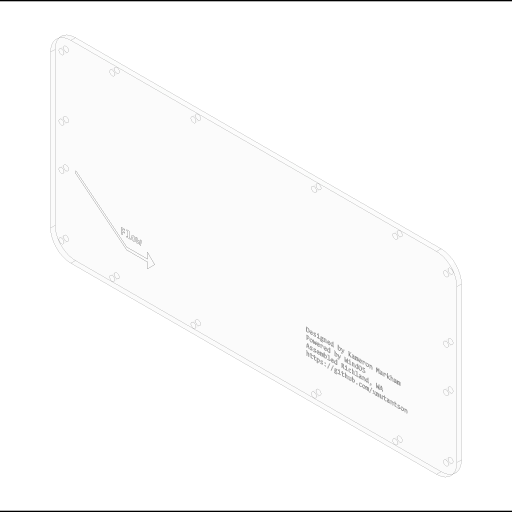
# Autodesk Inventor part: Wind Tunnel Test Section Door Outer
Saved by Autodesk Inventor 2023 (Build 270158000, 158)
## iProperties
Created: 2022-03-08
Part Number: Wind Tunnel Test Section Door Outer
Material: Polycarbonate, Clear
Document SubType Name: Modeling
Designer: kamer
Density: 1.2 g/cm^3
Appearance: Polycarbonate - Clear
Author: kamer
Autodesk Inventor part; units mm, degrees
(part 1 of 3)
ref_plane "YZ Plane" through (0, 0, 0) normal (1, 0, 0) x (0, 1, 0)
ref_plane "XZ Plane" through (0, 0, 0) normal (0, 1, 0) x (-1, 0, 0)
ref_plane "XY Plane" through (0, 0, 0) normal (0, 0, 1) x (1, 0, 0)
sketch "Sketch1" plane through (0, 0, 0) normal (0, 0, 1) x (1, 0, 0)
  line L0 (25.4, 0) -> (482.6, 0)
  line L1 (508, 25.4) -> (508, 215.9)
  line L2 (482.6, 241.3) -> (25.4, 241.3)
  line L3 (0, 215.9) -> (0, 25.4)
  arc A0 (25.4, 241.3) -> (0, 215.9) centre (25.4, 215.9) ccw
  arc A1 (508, 215.9) -> (482.6, 241.3) centre (482.6, 215.9) ccw
  arc A2 (482.6, 0) -> (508, 25.4) centre (482.6, 25.4) ccw
  arc A3 (0, 25.4) -> (25.4, 0) centre (25.4, 25.4) ccw
  point P0 (0, 0)
  point P1 (508, 241.3)
  point P2 (508, 0)
  point P3 (0, 241.3)
  dimension "d0" = 508
  dimension "d1" = 241.3
  dimension "d2" = 25.4
  constraints: 8 end point, 8 point on circle, 8 point on line, 8 tangent, 4 centre point, 3 equal radius, 2 parallel, 1 horizontal, 1 perpendicular
  measures "d0" distance of point (0, 241.3) point (508, 241.3)
  measures "d1" distance of point (508, 241.3) point (508, 0)
  measures "d2" radius of A0
extrude "Extrusion1" add sketch "Sketch1" along normal blind 5.7658
sketch "Sketch2" plane through (0, 0, 5.7658) normal (0, 0, 1) x (1, 0, 0)
  circle A0 centre (13.589, 223.012) radius 3.175
  line L0 (0, 215.9) -> (0, 25.4) projected
  line L1 (482.6, 241.3) -> (25.4, 241.3) projected
  circle A1 centre (13.589, 146.812) radius 3.175
  circle A2 centre (13.589, 94.4626) radius 3.175
  circle A3 centre (13.589, 18.2626) radius 3.175
  circle A4 centre (494.4364, 223.012) radius 3.175
  circle A5 centre (494.4364, 146.812) radius 3.175
  circle A6 centre (494.4364, 94.4626) radius 3.175
  circle A7 centre (494.4364, 18.2626) radius 3.175
  circle A8 centre (77.089, 231.902) radius 3.175
  circle A9 centre (178.689, 231.902) radius 3.175
  circle A10 centre (329.3364, 231.902) radius 3.175
  circle A11 centre (430.9364, 231.902) radius 3.175
  circle A12 centre (77.089, 9.3726) radius 3.175
  circle A13 centre (178.689, 9.3726) radius 3.175
  circle A14 centre (329.3364, 9.3726) radius 3.175
  circle A15 centre (430.9364, 9.3726) radius 3.175
  point P0 (0, 0)
  dimension "d5" = 6.35
  dimension "d6" = 13.589
  dimension "d7" = 18.288
  dimension "d8" = 6.35
  dimension "d9" = 76.2
  dimension "d10" = 13.589
  dimension "d11" = 6.35
  dimension "d12" = 52.3494
  dimension "d13" = 13.589
  dimension "d14" = 6.35
  dimension "d15" = 76.2
  dimension "d16" = 13.589
  dimension "d19" = 480.8474
  dimension "d24" = 6.35
  dimension "d25" = 63.5
  dimension "d26" = 8.89
  dimension "d27" = 6.35
  dimension "d28" = 101.6
  dimension "d29" = 6.35
  dimension "d30" = 150.6474
  dimension "d31" = 6.35
  dimension "d32" = 101.6
  dimension "d33" = 9.398
  dimension "d34" = 9.398
  dimension "d35" = 9.398
  dimension "d38" = 222.5294
  constraints: 16 centre point, 1 horizontal, 1 vertical, 16 other
  measures "d5" diameter of A0
  measures "d6" distance from line of L0 A0.centre
  measures "d7" distance from line of A0.centre L1
  measures "d8" diameter of A1
  measures "d9" distance of A1.centre A0.centre
  measures "d10" distance from line of L0 A1.centre
  measures "d11" diameter of A2
  measures "d12" distance of A2.centre A1.centre
  measures "d13" distance from line of L0 A2.centre
  measures "d14" diameter of A3
  measures "d15" distance of A3.centre A2.centre
  measures "d16" distance from line of L0 A3.centre
  measures "d19" distance of A0.centre A4.centre
  measures "d24" diameter of A8
  measures "d25" horizontal distance of A8.centre A0.centre
  measures "d26" vertical distance of A0.centre A8.centre
  measures "d27" diameter of A9
  measures "d28" distance of A9.centre A8.centre
  measures "d29" diameter of A10
  measures "d30" distance of A10.centre A9.centre
  measures "d31" diameter of A11
  measures "d32" distance of A10.centre A11.centre
  measures "d33" distance from line of L1 A11.centre
  measures "d34" distance from line of L1 A10.centre
  measures "d35" distance from line of L1 A9.centre
  measures "d38" distance of A8.centre A12.centre
extrude "Extrusion2" cut sketch "Sketch2" against normal through all
sketch "Sketch3" plane through (0, 0, 5.7658) normal (0, 0, 1) x (1, 0, 0)
  line L0 (31.75, 101.6) -> (95.25, 50.8) construction
  line L1 (95.25, 50.8) -> (121.1904, 50.8) construction
  line L2 (130.175, 50.8) -> (121.1904, 59.7846)
  line L3 (121.1904, 59.7846) -> (121.1904, 41.8154)
  line L4 (121.1904, 41.8154) -> (130.175, 50.8)
  line L5 (0, 215.9) -> (0, 25.4) projected
  line L6 (25.4, 0) -> (482.6, 0) projected
  line L7 (87.4073, 71.1521) -> (112.3915, 71.1521) construction
  line L8 (112.3915, 71.1521) -> (112.3915, 60.7928) construction
  line L9 (112.3915, 60.7928) -> (87.4073, 60.7928) construction
  line L10 (87.4073, 60.7928) -> (87.4073, 71.1521) construction
  line L11 (319.3804, 78.7378) -> (430.3775, 78.7378) construction
  line L12 (430.3775, 78.7378) -> (430.3775, 29.4798) construction
  line L13 (430.3775, 29.4798) -> (319.3804, 29.4798) construction
  line L14 (319.3804, 29.4798) -> (319.3804, 78.7378) construction
  line L15 (121.1904, 52.3875) -> (95.2986, 52.3875)
  line L16 (95.2986, 52.3875) -> (31.731, 103.2416)
  line L17 (121.1904, 49.2125) -> (95.2014, 49.2125)
  line L18 (95.2014, 49.2125) -> (31.731, 99.9888)
  line L19 (31.731, 99.9888) -> (31.731, 103.2416)
  line L20 (89.9405, 69.3154) -> (89.9405, 67.2124)
  line L21 (89.9405, 67.2124) -> (92.8151, 67.2124)
  line L22 (92.8151, 67.2124) -> (92.8151, 66.0312)
  line L23 (92.8151, 66.0312) -> (89.9405, 66.0312)
  line L24 (89.9405, 66.0312) -> (89.9405, 62.9108)
  line L25 (89.9405, 62.9108) -> (88.4793, 62.9108)
  line L26 (88.4793, 62.9108) -> (88.4793, 70.5308)
  line L27 (88.4793, 70.5308) -> (92.9789, 70.5308)
  line L28 (92.9789, 70.5308) -> (92.9789, 69.3154)
  line L29 (92.9789, 69.3154) -> (89.9405, 69.3154)
  line L30 (96.7002, 70.046) -> (95.0341, 70.046)
  line L31 (95.0341, 70.046) -> (95.0341, 71.1521)
  line L32 (95.0341, 71.1521) -> (98.1613, 71.1521)
  line L33 (98.1613, 71.1521) -> (98.1613, 64.0169)
  line L34 (98.1613, 64.0169) -> (99.8683, 64.0169)
  line L35 (99.8683, 64.0169) -> (99.8683, 62.9108)
  line L36 (99.8683, 62.9108) -> (94.8293, 62.9108)
  line L37 (94.8293, 62.9108) -> (94.8293, 64.0169)
  line L38 (94.8293, 64.0169) -> (96.7002, 64.0169)
  line L39 (96.7002, 64.0169) -> (96.7002, 70.046)
  spline S0 degree 2 poles (106.6895, 65.9151) (106.6895, 65.2186) (106.2934, 64.0579) (105.5492, 63.2317) (104.4636, 62.7742) (103.7671, 62.7742) knots 0 0 0 1 2 3 4 4 4
  spline S1 degree 2 poles (103.7671, 62.7742) (103.1048, 62.7742) (102.0669, 63.1566) (101.3432, 63.9213) (100.9608, 65.0684) (100.9608, 65.8331) knots 0 0 0 1 2 3 4 4 4
  spline S2 degree 2 poles (100.9608, 65.8331) (100.9608, 66.5433) (101.3637, 67.6972) (102.1147, 68.5097) (103.2004, 68.9603) (103.8832, 68.9603) knots 0 0 0 1 2 3 4 4 4
  spline S3 degree 2 poles (103.8832, 68.9603) (104.5455, 68.9603) (105.5902, 68.5712) (106.3071, 67.7996) (106.6895, 66.6662) (106.6895, 65.9151) knots 0 0 0 1 2 3 4 4 4
  spline S4 degree 2 poles (105.2078, 65.8809) (105.2078, 66.8027) (104.5113, 67.7313) (103.8354, 67.7313) knots 0 0 0 1 2 2 2
  spline S5 degree 2 poles (103.8354, 67.7313) (103.4667, 67.7313) (102.9409, 67.4377) (102.5995, 66.9324) (102.4425, 66.2565) (102.4425, 65.8673) knots 0 0 0 1 2 3 4 4 4
  spline S6 degree 2 poles (102.4425, 65.8673) (102.4425, 64.9455) (103.1867, 64.0033) (103.8354, 64.0033) knots 0 0 0 1 2 2 2
  spline S7 degree 2 poles (103.8354, 64.0033) (104.1904, 64.0033) (104.7162, 64.29) (105.0439, 64.7953) (105.2078, 65.4849) (105.2078, 65.8809) knots 0 0 0 1 2 3 4 4 4
  line L40 (112.7868, 62.9108) -> (111.2096, 62.9108)
  line L41 (111.2096, 62.9108) -> (110.5814, 64.7953)
  line L42 (110.5814, 64.7953) -> (110.3902, 65.4508)
  line L43 (110.3902, 65.4508) -> (110.1922, 64.7748)
  line L44 (110.1922, 64.7748) -> (109.5845, 62.9108)
  line L45 (109.5845, 62.9108) -> (108.0004, 62.9108)
  line L46 (108.0004, 62.9108) -> (107.1674, 68.8374)
  line L47 (107.1674, 68.8374) -> (108.5194, 68.8374)
  line L48 (108.5194, 68.8374) -> (108.9427, 65.4781)
  line L49 (108.9427, 65.4781) -> (109.0383, 64.57)
  line L50 (109.0383, 64.57) -> (109.2773, 65.3962)
  line L51 (109.2773, 65.3962) -> (109.8713, 67.1987)
  line L52 (109.8713, 67.1987) -> (110.9569, 67.1987)
  line L53 (110.9569, 67.1987) -> (111.5919, 65.403)
  line L54 (111.5919, 65.403) -> (111.8651, 64.5563)
  line L55 (111.8651, 64.5563) -> (111.9743, 65.4986)
  line L56 (111.9743, 65.4986) -> (112.3362, 68.8374)
  line L57 (112.3362, 68.8374) -> (113.6267, 68.8374)
  line L58 (113.6267, 68.8374) -> (112.7868, 62.9108)
  spline S8 degree 2 poles (323.4726, 75.7927) (323.4726, 75.4285) (323.3588, 74.7594) (323.113, 74.1858) (322.717, 73.717) (322.1389, 73.3801) (321.3787, 73.1981) (320.8916, 73.1981) knots 0 0 0 1 2 3 4 5 6 6 6
  line L59 (320.8916, 73.1981) -> (319.8037, 73.1981)
  line L60 (319.8037, 73.1981) -> (319.8037, 78.2781)
  line L61 (319.8037, 78.2781) -> (321.1147, 78.2781)
  spline S9 degree 2 poles (321.1147, 78.2781) (322.3028, 78.2781) (323.4726, 77.0536) (323.4726, 75.7927) knots 0 0 0 1 2 2 2
  spline S10 degree 2 poles (322.7443, 75.7472) (322.7443, 76.2843) (322.544, 77.0308) (322.1298, 77.4906) (321.5107, 77.6954) (321.0919, 77.6954) knots 0 0 0 1 2 3 4 4 4
  line L62 (321.0919, 77.6954) -> (320.4956, 77.6954)
  line L63 (320.4956, 77.6954) -> (320.4956, 73.7989)
  line L64 (320.4956, 73.7989) -> (321.01, 73.7989)
  spline S11 degree 2 poles (321.01, 73.7989) (322.7443, 73.7989) (322.7443, 75.7472) knots 0 0 0 1 1 1
  spline S12 degree 2 poles (327.6786, 75.3557) (327.6786, 75.2146) (327.6695, 75.0188) (327.665, 74.9324) knots 0 0 0 1 2 2 2
  line L65 (327.665, 74.9324) -> (324.9201, 74.9324)
  spline S13 degree 2 poles (324.9201, 74.9324) (324.9201, 74.336) (325.5893, 73.6942) (326.222, 73.6942) knots 0 0 0 1 2 2 2
  spline S14 degree 2 poles (326.222, 73.6942) (326.3904, 73.6942) (326.7318, 73.7215) (327.055, 73.7671) (327.3463, 73.8262) (327.4692, 73.8626) knots 0 0 0 1 2 3 4 4 4
  line L66 (327.4692, 73.8626) -> (327.4692, 73.3073)
  spline S15 degree 2 poles (327.4692, 73.3073) (327.1916, 73.2299) (326.4951, 73.1298) (326.1219, 73.1298) knots 0 0 0 1 2 2 2
  spline S16 degree 2 poles (326.1219, 73.1298) (325.6211, 73.1298) (324.8974, 73.4029) (324.4376, 73.9173) (324.2146, 74.6683) (324.2146, 75.1417) knots 0 0 0 1 2 3 4 4 4
  spline S17 degree 2 poles (324.2146, 75.1417) (324.2146, 75.556) (324.4513, 76.2888) (324.9065, 76.8442) (325.5665, 77.1719) (325.9853, 77.1719) knots 0 0 0 1 2 3 4 4 4
  spline S18 degree 2 poles (325.9853, 77.1719) (326.395, 77.1719) (327.0277, 76.917) (327.4556, 76.4436) (327.6786, 75.7745) (327.6786, 75.3557) knots 0 0 0 1 2 3 4 4 4
  spline S19 degree 2 poles (326.9731, 75.4513) (326.9867, 75.7107) (326.8593, 76.1432) (326.5998, 76.4573) (326.2129, 76.6302) (325.9534, 76.6302) knots 0 0 0 1 2 3 4 4 4
  spline S20 degree 2 poles (325.9534, 76.6302) (325.7349, 76.6302) (325.3662, 76.4573) (325.1022, 76.1477) (324.9384, 75.7107) (324.9201, 75.4513) knots 0 0 0 1 2 3 4 4 4
  line L67 (324.9201, 75.4513) -> (326.9731, 75.4513)
  spline S21 degree 2 poles (331.8482, 74.2632) (331.8482, 74.0584) (331.7071, 73.7306) (331.4659, 73.4803) (331.1472, 73.3028) (330.7876, 73.1844) (330.4053, 73.1298) (330.2232, 73.1298) knots 0 0 0 1 2 3 4 5 6 6 6
  spline S22 degree 2 poles (330.2232, 73.1298) (329.8272, 73.1298) (329.1626, 73.2026) (328.8439, 73.28) knots 0 0 0 1 2 2 2
  line L68 (328.8439, 73.28) -> (328.8439, 73.9036)
  spline S23 degree 2 poles (328.8439, 73.9036) (329.1853, 73.8035) (329.8636, 73.7033) (330.1959, 73.7033) knots 0 0 0 1 2 2 2
  spline S24 degree 2 poles (330.1959, 73.7033) (330.6829, 73.7033) (331.1472, 73.9673) (331.1472, 74.2086) knots 0 0 0 1 2 2 2
  spline S25 degree 2 poles (331.1472, 74.2086) (331.1472, 74.3133) (331.0744, 74.4817) (330.8787, 74.6319) (330.4735, 74.7958) (330.1185, 74.9005) knots 0 0 0 1 2 3 4 4 4
  spline S26 degree 2 poles (330.1185, 74.9005) (329.8545, 74.9779) (329.4084, 75.1782) (329.0806, 75.4513) (328.894, 75.8154) (328.894, 76.0658) knots 0 0 0 1 2 3 4 4 4
  spline S27 degree 2 poles (328.894, 76.0658) (328.894, 76.2297) (329.0442, 76.6166) (329.4129, 76.9489) (330.032, 77.1719) (330.5009, 77.1719) knots 0 0 0 1 2 3 4 4 4
  spline S28 degree 2 poles (330.5009, 77.1719) (330.7285, 77.1719) (331.2884, 77.1219) (331.5933, 77.0581) knots 0 0 0 1 2 2 2
  line L69 (331.5933, 77.0581) -> (331.5933, 76.4573)
  spline S29 degree 2 poles (331.5933, 76.4573) (331.2747, 76.5347) (330.7011, 76.6075) (330.4918, 76.6075) knots 0 0 0 1 2 2 2
  spline S30 degree 2 poles (330.4918, 76.6075) (330.2414, 76.6075) (329.8954, 76.5301) (329.6815, 76.3935) (329.5859, 76.2115) (329.5859, 76.1068) knots 0 0 0 1 2 3 4 4 4
  spline S31 degree 2 poles (329.5859, 76.1068) (329.5859, 76.0021) (329.6679, 75.8291) (329.8909, 75.6698) (330.2869, 75.5105) (330.6056, 75.4194) knots 0 0 0 1 2 3 4 4 4
  spline S32 degree 2 poles (330.6056, 75.4194) (330.9515, 75.3193) (331.4249, 75.0962) (331.7208, 74.8231) (331.8482, 74.4817) (331.8482, 74.2632) knots 0 0 0 1 2 3 4 4 4
  line L70 (334.4702, 76.5392) -> (333.314, 76.5392)
  line L71 (333.314, 76.5392) -> (333.314, 77.0991)
  line L72 (333.314, 77.0991) -> (335.153, 77.0991)
  line L73 (335.153, 77.0991) -> (335.153, 73.7625)
  line L74 (335.153, 73.7625) -> (336.3137, 73.7625)
  line L75 (336.3137, 73.7625) -> (336.3137, 73.1981)
  line L76 (336.3137, 73.1981) -> (333.1865, 73.1981)
  line L77 (333.1865, 73.1981) -> (333.1865, 73.7625)
  line L78 (333.1865, 73.7625) -> (334.4702, 73.7625)
  line L79 (334.4702, 73.7625) -> (334.4702, 76.5392)
  spline S33 degree 2 poles (334.7069, 78.7378) (334.8207, 78.7378) (335.0119, 78.6559) (335.1575, 78.5102) (335.2395, 78.319) (335.2395, 78.2052) knots 0 0 0 1 2 3 4 4 4
  spline S34 degree 2 poles (335.2395, 78.2052) (335.2395, 78.096) (335.1575, 77.9002) (335.0119, 77.7546) (334.8207, 77.6726) (334.7069, 77.6726) knots 0 0 0 1 2 3 4 4 4
  spline S35 degree 2 poles (334.7069, 77.6726) (334.5931, 77.6726) (334.4019, 77.7546) (334.2562, 77.9002) (334.1743, 78.096) (334.1743, 78.2052) knots 0 0 0 1 2 3 4 4 4
  spline S36 degree 2 poles (334.1743, 78.2052) (334.1743, 78.319) (334.2562, 78.5102) (334.4019, 78.6559) (334.5931, 78.7378) (334.7069, 78.7378) knots 0 0 0 1 2 3 4 4 4
  spline S37 degree 2 poles (340.3286, 76.5483) (340.4378, 76.4117) (340.5562, 76.0521) (340.5562, 75.8428) knots 0 0 0 1 2 2 2
  spline S38 degree 2 poles (340.5562, 75.8428) (340.5562, 75.5378) (340.3331, 75.0371) (339.9325, 74.682) (339.3681, 74.4817) (339.0313, 74.4817) knots 0 0 0 1 2 3 4 4 4
  spline S39 degree 2 poles (339.0313, 74.4817) (338.7854, 74.4817) (338.3576, 74.5864) (338.2347, 74.6638) knots 0 0 0 1 2 2 2
  spline S40 degree 2 poles (338.2347, 74.6638) (338.1573, 74.5545) (338.0571, 74.3634) (338.0571, 74.2405) knots 0 0 0 1 2 2 2
  spline S41 degree 2 poles (338.0571, 74.2405) (338.0571, 74.0948) (338.3394, 73.8991) (338.5761, 73.89) knots 0 0 0 1 2 2 2
  line L80 (338.5761, 73.89) -> (339.6003, 73.8535)
  spline S42 degree 2 poles (339.6003, 73.8535) (339.8916, 73.8444) (340.3877, 73.7124) (340.7382, 73.4621) (340.9385, 73.0979) (340.9385, 72.8567) knots 0 0 0 1 2 3 4 4 4
  spline S43 degree 2 poles (340.9385, 72.8567) (340.9385, 72.5972) (340.7109, 72.1283) (340.2421, 71.7733) (339.5183, 71.5639) (339.0222, 71.5639) knots 0 0 0 1 2 3 4 4 4
  spline S44 degree 2 poles (339.0222, 71.5639) (338.5487, 71.5639) (337.8842, 71.7141) (337.4563, 71.9827) (337.2605, 72.3514) (337.2605, 72.5744) knots 0 0 0 1 2 3 4 4 4
  spline S45 degree 2 poles (337.2605, 72.5744) (337.2605, 72.8612) (337.5246, 73.2891) (337.8022, 73.4848) knots 0 0 0 1 2 2 2
  spline S46 degree 2 poles (337.8022, 73.4848) (337.6975, 73.5303) (337.5519, 73.6715) (337.4563, 73.8399) (337.4108, 74.0265) (337.4108, 74.1176) knots 0 0 0 1 2 3 4 4 4
  spline S47 degree 2 poles (337.4108, 74.1176) (337.4108, 74.3679) (337.6475, 74.7867) (337.8113, 74.9733) knots 0 0 0 1 2 2 2
  spline S48 degree 2 poles (337.8113, 74.9733) (337.7385, 75.0644) (337.6247, 75.2373) (337.5428, 75.4331) (337.5018, 75.6652) (337.5018, 75.8109) knots 0 0 0 1 2 3 4 4 4
  spline S49 degree 2 poles (337.5018, 75.8109) (337.5018, 76.1159) (337.7248, 76.6166) (338.1254, 76.9716) (338.6853, 77.1719) (339.0267, 77.1719) knots 0 0 0 1 2 3 4 4 4
  spline S50 degree 2 poles (339.0267, 77.1719) (339.1724, 77.1719) (339.4364, 77.131) (339.5365, 77.0991) knots 0 0 0 1 2 2 2
  line L81 (339.5365, 77.0991) -> (340.9522, 77.0991)
  line L82 (340.9522, 77.0991) -> (340.9522, 76.5483)
  line L83 (340.9522, 76.5483) -> (340.3286, 76.5483)
  spline S51 degree 2 poles (338.1846, 75.8291) (338.1846, 75.6425) (338.3075, 75.3284) (338.5351, 75.1099) (338.8401, 74.9915) (339.0313, 74.9915) knots 0 0 0 1 2 3 4 4 4
  spline S52 degree 2 poles (339.0313, 74.9915) (339.2315, 74.9915) (339.5456, 75.1281) (339.7596, 75.3602) (339.8734, 75.6652) (339.8734, 75.8291) knots 0 0 0 1 2 3 4 4 4
  spline S53 degree 2 poles (339.8734, 75.8291) (339.8734, 76.0112) (339.7505, 76.3253) (339.5229, 76.5438) (339.2179, 76.6621) (339.0313, 76.6621) knots 0 0 0 1 2 3 4 4 4
  spline S54 degree 2 poles (339.0313, 76.6621) (338.8264, 76.6621) (338.5123, 76.521) (338.2984, 76.2934) (338.1846, 75.9884) (338.1846, 75.8291) knots 0 0 0 1 2 3 4 4 4
  spline S55 degree 2 poles (337.9798, 72.6336) (337.9798, 72.3605) (338.5533, 72.1056) (339.0677, 72.1056) knots 0 0 0 1 2 2 2
  spline S56 degree 2 poles (339.0677, 72.1056) (339.3909, 72.1056) (339.8279, 72.2239) (340.0964, 72.4106) (340.2148, 72.6564) (340.2148, 72.7838) knots 0 0 0 1 2 3 4 4 4
  spline S57 degree 2 poles (340.2148, 72.7838) (340.2148, 73.0205) (339.8279, 73.2481) (339.4273, 73.2663) knots 0 0 0 1 2 2 2
  line L84 (339.4273, 73.2663) -> (338.4076, 73.3028)
  spline S58 degree 2 poles (338.4076, 73.3028) (338.2802, 73.2163) (338.1118, 73.0524) (338.0207, 72.8885) (337.9798, 72.7201) (337.9798, 72.6336) knots 0 0 0 1 2 3 4 4 4
  line L85 (341.899, 77.0991) -> (342.5044, 77.0991)
  line L86 (342.5044, 77.0991) -> (342.5317, 76.4709)
  spline S59 degree 2 poles (342.5317, 76.4709) (342.7001, 76.6712) (343.0188, 76.9398) (343.3283, 77.1036) (343.647, 77.1719) (343.8199, 77.1719) knots 0 0 0 1 2 3 4 4 4
  spline S60 degree 2 poles (343.8199, 77.1719) (344.4208, 77.1719) (345.0399, 76.4618) (345.0399, 75.7472) knots 0 0 0 1 2 2 2
  line L87 (345.0399, 75.7472) -> (345.0399, 73.1981)
  line L88 (345.0399, 73.1981) -> (344.3616, 73.1981)
  line L89 (344.3616, 73.1981) -> (344.3616, 75.6925)
  spline S61 degree 2 poles (344.3616, 75.6925) (344.3616, 76.1477) (344.0202, 76.5893) (343.6834, 76.5893) knots 0 0 0 1 2 2 2
  spline S62 degree 2 poles (343.6834, 76.5893) (343.5559, 76.5893) (343.3192, 76.5164) (343.0643, 76.3344) (342.7639, 76.0203) (342.5772, 75.7881) knots 0 0 0 1 2 3 4 4 4
  line L90 (342.5772, 75.7881) -> (342.5772, 73.1981)
  line L91 (342.5772, 73.1981) -> (341.899, 73.1981)
  line L92 (341.899, 73.1981) -> (341.899, 77.0991)
  spline S63 degree 2 poles (349.5736, 75.3557) (349.5736, 75.2146) (349.5645, 75.0188) (349.56, 74.9324) knots 0 0 0 1 2 2 2
  line L93 (349.56, 74.9324) -> (346.8151, 74.9324)
  spline S64 degree 2 poles (346.8151, 74.9324) (346.8151, 74.336) (347.4843, 73.6942) (348.117, 73.6942) knots 0 0 0 1 2 2 2
  spline S65 degree 2 poles (348.117, 73.6942) (348.2854, 73.6942) (348.6268, 73.7215) (348.95, 73.7671) (349.2413, 73.8262) (349.3642, 73.8626) knots 0 0 0 1 2 3 4 4 4
  line L94 (349.3642, 73.8626) -> (349.3642, 73.3073)
  spline S66 degree 2 poles (349.3642, 73.3073) (349.0866, 73.2299) (348.3901, 73.1298) (348.0168, 73.1298) knots 0 0 0 1 2 2 2
  spline S67 degree 2 poles (348.0168, 73.1298) (347.5161, 73.1298) (346.7924, 73.4029) (346.3326, 73.9173) (346.1096, 74.6683) (346.1096, 75.1417) knots 0 0 0 1 2 3 4 4 4
  spline S68 degree 2 poles (346.1096, 75.1417) (346.1096, 75.556) (346.3463, 76.2888) (346.8015, 76.8442) (347.4615, 77.1719) (347.8803, 77.1719) knots 0 0 0 1 2 3 4 4 4
  spline S69 degree 2 poles (347.8803, 77.1719) (348.29, 77.1719) (348.9227, 76.917) (349.3506, 76.4436) (349.5736, 75.7745) (349.5736, 75.3557) knots 0 0 0 1 2 3 4 4 4
  spline S70 degree 2 poles (348.8681, 75.4513) (348.8817, 75.7107) (348.7543, 76.1432) (348.4948, 76.4573) (348.1079, 76.6302) (347.8484, 76.6302) knots 0 0 0 1 2 3 4 4 4
  spline S71 degree 2 poles (347.8484, 76.6302) (347.6299, 76.6302) (347.2612, 76.4573) (346.9972, 76.1477) (346.8333, 75.7107) (346.8151, 75.4513) knots 0 0 0 1 2 3 4 4 4
  line L95 (346.8151, 75.4513) -> (348.8681, 75.4513)
  spline S72 degree 2 poles (350.4567, 75.0689) (350.4567, 75.5651) (350.7298, 76.3389) (351.2305, 76.8715) (351.9315, 77.1492) (352.364, 77.1492) knots 0 0 0 1 2 3 4 4 4
  spline S73 degree 2 poles (352.364, 77.1492) (352.5506, 77.1492) (352.9148, 77.1036) (353.0877, 77.0536) knots 0 0 0 1 2 2 2
  line L96 (353.0877, 77.0536) -> (353.0877, 78.6923)
  line L97 (353.0877, 78.6923) -> (353.766, 78.6923)
  line L98 (353.766, 78.6923) -> (353.766, 73.1981)
  line L99 (353.766, 73.1981) -> (353.1606, 73.1981)
  line L100 (353.1606, 73.1981) -> (353.1378, 73.94)
  spline S74 degree 2 poles (353.1378, 73.94) (352.8556, 73.5258) (352.1956, 73.1298) (351.8086, 73.1298) knots 0 0 0 1 2 2 2
  spline S75 degree 2 poles (351.8086, 73.1298) (351.4763, 73.1298) (350.9665, 73.4074) (350.6297, 73.9173) (350.4567, 74.6319) (350.4567, 75.0689) knots 0 0 0 1 2 3 4 4 4
  spline S76 degree 2 poles (351.1486, 75.1099) (351.1486, 74.4043) (351.5628, 73.7079) (351.9452, 73.7079) knots 0 0 0 1 2 2 2
  spline S77 degree 2 poles (351.9452, 73.7079) (352.2001, 73.7079) (352.7737, 74.1676) (353.0877, 74.6183) knots 0 0 0 1 2 2 2
  line L101 (353.0877, 74.6183) -> (353.0877, 76.43)
  spline S78 degree 2 poles (353.0877, 76.43) (352.9193, 76.5073) (352.5187, 76.5893) (352.3185, 76.5893) knots 0 0 0 1 2 2 2
  spline S79 degree 2 poles (352.3185, 76.5893) (351.7677, 76.5893) (351.1486, 75.8746) (351.1486, 75.1099) knots 0 0 0 1 2 2 2
  spline S80 degree 2 poles (362.7516, 75.2191) (362.7516, 74.7366) (362.483, 73.9673) (361.9914, 73.4348) (361.2813, 73.1525) (360.8398, 73.1525) knots 0 0 0 1 2 3 4 4 4
  spline S81 degree 2 poles (360.8398, 73.1525) (360.4938, 73.1525) (359.77, 73.2845) (359.415, 73.4302) knots 0 0 0 1 2 2 2
  line L102 (359.415, 73.4302) -> (359.415, 78.6923)
  line L103 (359.415, 78.6923) -> (360.0932, 78.6923)
  line L104 (360.0932, 78.6923) -> (360.0932, 77.181)
  line L105 (360.0932, 77.181) -> (360.0614, 76.4573)
  spline S82 degree 2 poles (360.0614, 76.4573) (360.3527, 76.8487) (361.0173, 77.1719) (361.3996, 77.1719) knots 0 0 0 1 2 2 2
  spline S83 degree 2 poles (361.3996, 77.1719) (361.7319, 77.1719) (362.2372, 76.8943) (362.5786, 76.3844) (362.7516, 75.6652) (362.7516, 75.2191) knots 0 0 0 1 2 3 4 4 4
  spline S84 degree 2 poles (362.0597, 75.1873) (362.0597, 75.4968) (361.9686, 76.0066) (361.7775, 76.3753) (361.4725, 76.5802) (361.2631, 76.5802) knots 0 0 0 1 2 3 4 4 4
  spline S85 degree 2 poles (361.2631, 76.5802) (361.1356, 76.5802) (360.8716, 76.4982) (360.5848, 76.3071) (360.2708, 75.993) (360.0932, 75.7608) knots 0 0 0 1 2 3 4 4 4
  line L106 (360.0932, 75.7608) -> (360.0932, 73.8672)
  spline S86 degree 2 poles (360.0932, 73.8672) (360.2935, 73.7898) (360.7032, 73.6988) (360.8898, 73.6988) knots 0 0 0 1 2 2 2
  spline S87 degree 2 poles (360.8898, 73.6988) (361.122, 73.6988) (361.5453, 73.8444) (361.8685, 74.1904) (362.0597, 74.7639) (362.0597, 75.1873) knots 0 0 0 1 2 3 4 4 4
  line L107 (367.2671, 77.0991) -> (365.938, 73.6123)
  spline S88 degree 2 poles (365.938, 73.6123) (365.7286, 73.0797) (365.2916, 72.3104) (364.7681, 71.8143) (364.149, 71.5821) (363.7621, 71.5821) knots 0 0 0 1 2 3 4 4 4
  spline S89 degree 2 poles (363.7621, 71.5821) (363.662, 71.5821) (363.4981, 71.5912) (363.4025, 71.6003) knots 0 0 0 1 2 2 2
  line L108 (363.4025, 71.6003) -> (363.4025, 72.2148)
  spline S90 degree 2 poles (363.4025, 72.2148) (363.4844, 72.2012) (363.6893, 72.183) (363.8031, 72.183) knots 0 0 0 1 2 2 2
  spline S91 degree 2 poles (363.8031, 72.183) (363.9897, 72.183) (364.3129, 72.2922) (364.5997, 72.5335) (364.8637, 72.9249) (364.9866, 73.1981) knots 0 0 0 1 2 3 4 4 4
  line L109 (364.9866, 73.1981) -> (363.4298, 77.0991)
  line L110 (363.4298, 77.0991) -> (364.1991, 77.0991)
  line L111 (364.1991, 77.0991) -> (365.1869, 74.5181)
  line L112 (365.1869, 74.5181) -> (365.3872, 73.9127)
  line L113 (365.3872, 73.9127) -> (365.6102, 74.5363)
  line L114 (365.6102, 74.5363) -> (366.5206, 77.0991)
  line L115 (366.5206, 77.0991) -> (367.2671, 77.0991)
  line L116 (375.9978, 73.1981) -> (375.1284, 73.1981)
  line L117 (375.1284, 73.1981) -> (373.2257, 75.688)
  line L118 (373.2257, 75.688) -> (373.2257, 73.1981)
  line L119 (373.2257, 73.1981) -> (372.5338, 73.1981)
  line L120 (372.5338, 73.1981) -> (372.5338, 78.2781)
  line L121 (372.5338, 78.2781) -> (373.2257, 78.2781)
  line L122 (373.2257, 78.2781) -> (373.2257, 75.9156)
  line L123 (373.2257, 75.9156) -> (375.0874, 78.2781)
  line L124 (375.0874, 78.2781) -> (375.9068, 78.2781)
  line L125 (375.9068, 78.2781) -> (373.9039, 75.8655)
  line L126 (373.9039, 75.8655) -> (375.9978, 73.1981)
  line L127 (379.4391, 73.1981) -> (379.4255, 73.7215)
  spline S92 degree 2 poles (379.4255, 73.7215) (379.1068, 73.4074) (378.4468, 73.1298) (378.0872, 73.1298) knots 0 0 0 1 2 2 2
  spline S93 degree 2 poles (378.0872, 73.1298) (377.7503, 73.1298) (377.2769, 73.3028) (376.9719, 73.5986) (376.8263, 74.0038) (376.8263, 74.2405) knots 0 0 0 1 2 3 4 4 4
  spline S94 degree 2 poles (376.8263, 74.2405) (376.8263, 74.8277) (377.7003, 75.4922) (378.556, 75.4922) knots 0 0 0 1 2 2 2
  line L128 (378.556, 75.4922) -> (379.3663, 75.4922)
  line L129 (379.3663, 75.4922) -> (379.3663, 75.8336)
  spline S95 degree 2 poles (379.3663, 75.8336) (379.3663, 76.1796) (378.9247, 76.5984) (378.4695, 76.5984) knots 0 0 0 1 2 2 2
  spline S96 degree 2 poles (378.4695, 76.5984) (378.1372, 76.5984) (377.4954, 76.4527) (377.154, 76.3162) knots 0 0 0 1 2 2 2
  line L130 (377.154, 76.3162) -> (377.154, 76.9261)
  spline S97 degree 2 poles (377.154, 76.9261) (377.2815, 76.9716) (377.5956, 77.0627) (377.9461, 77.131) (378.3284, 77.1719) (378.5196, 77.1719) knots 0 0 0 1 2 3 4 4 4
  spline S98 degree 2 poles (378.5196, 77.1719) (378.8747, 77.1719) (379.4437, 77.0172) (379.8351, 76.6985) (380.0445, 76.216) (380.0445, 75.8883) knots 0 0 0 1 2 3 4 4 4
  line L131 (380.0445, 75.8883) -> (380.0445, 73.1981)
  line L132 (380.0445, 73.1981) -> (379.4391, 73.1981)
  line L133 (379.3663, 74.9733) -> (378.506, 74.9733)
  spline S99 degree 2 poles (378.506, 74.9733) (378.251, 74.9733) (377.8869, 74.8732) (377.6547, 74.6865) (377.5409, 74.4271) (377.5409, 74.2632) knots 0 0 0 1 2 3 4 4 4
  spline S100 degree 2 poles (377.5409, 74.2632) (377.5409, 74.1494) (377.6092, 73.9446) (377.7685, 73.7853) (378.0143, 73.6942) (378.1964, 73.6942) knots 0 0 0 1 2 3 4 4 4
  spline S101 degree 2 poles (378.1964, 73.6942) (378.4286, 73.6942) (379.0294, 73.9764) (379.3663, 74.2814) knots 0 0 0 1 2 2 2
  line L134 (379.3663, 74.2814) -> (379.3663, 74.9733)
  line L135 (384.0958, 73.1981) -> (384.0958, 76.0021)
  spline S102 degree 2 poles (384.0958, 76.0021) (384.0958, 76.1841) (384.0685, 76.4163) (384.0138, 76.5529) (383.9319, 76.6075) (383.8682, 76.6075) knots 0 0 0 1 2 3 4 4 4
  spline S103 degree 2 poles (383.8682, 76.6075) (383.7953, 76.6075) (383.6724, 76.5164) (383.5313, 76.3025) (383.3629, 75.9565) (383.2446, 75.7062) knots 0 0 0 1 2 3 4 4 4
  line L136 (383.2446, 75.7062) -> (383.2446, 73.1981)
  line L137 (383.2446, 73.1981) -> (382.5663, 73.1981)
  line L138 (382.5663, 73.1981) -> (382.5663, 75.9292)
  spline S104 degree 2 poles (382.5663, 75.9292) (382.5663, 76.1432) (382.539, 76.4072) (382.4844, 76.5529) (382.3979, 76.6075) (382.3342, 76.6075) knots 0 0 0 1 2 3 4 4 4
  spline S105 degree 2 poles (382.3342, 76.6075) (382.2704, 76.6075) (382.1521, 76.5301) (382.011, 76.3298) (381.8334, 75.9793) (381.7151, 75.7062) knots 0 0 0 1 2 3 4 4 4
  line L139 (381.7151, 75.7062) -> (381.7151, 73.1981)
  line L140 (381.7151, 73.1981) -> (381.0368, 73.1981)
  line L141 (381.0368, 73.1981) -> (381.0368, 77.0991)
  line L142 (381.0368, 77.0991) -> (381.6013, 77.0991)
  line L143 (381.6013, 77.0991) -> (381.6332, 76.3571)
  spline S106 degree 2 poles (381.6332, 76.3571) (381.7379, 76.5802) (381.929, 76.8897) (382.1293, 77.0809) (382.3615, 77.1719) (382.498, 77.1719) knots 0 0 0 1 2 3 4 4 4
  spline S107 degree 2 poles (382.498, 77.1719) (382.8167, 77.1719) (383.1444, 76.7577) (383.1444, 76.3253) knots 0 0 0 1 2 2 2
  spline S108 degree 2 poles (383.1444, 76.3253) (383.2355, 76.5301) (383.4175, 76.8442) (383.6224, 77.0581) (383.8727, 77.1719) (384.0366, 77.1719) knots 0 0 0 1 2 3 4 4 4
  spline S109 degree 2 poles (384.0366, 77.1719) (384.774, 77.1719) (384.774, 76.0385) knots 0 0 0 1 1 1
  line L144 (384.774, 76.0385) -> (384.774, 73.1981)
  line L145 (384.774, 73.1981) -> (384.0958, 73.1981)
  spline S110 degree 2 poles (388.9846, 75.3557) (388.9846, 75.2146) (388.9755, 75.0188) (388.9709, 74.9324) knots 0 0 0 1 2 2 2
  line L146 (388.9709, 74.9324) -> (386.2261, 74.9324)
  spline S111 degree 2 poles (386.2261, 74.9324) (386.2261, 74.336) (386.8952, 73.6942) (387.528, 73.6942) knots 0 0 0 1 2 2 2
  spline S112 degree 2 poles (387.528, 73.6942) (387.6964, 73.6942) (388.0378, 73.7215) (388.361, 73.7671) (388.6523, 73.8262) (388.7752, 73.8626) knots 0 0 0 1 2 3 4 4 4
  line L147 (388.7752, 73.8626) -> (388.7752, 73.3073)
  spline S113 degree 2 poles (388.7752, 73.3073) (388.4975, 73.2299) (387.8011, 73.1298) (387.4278, 73.1298) knots 0 0 0 1 2 2 2
  spline S114 degree 2 poles (387.4278, 73.1298) (386.9271, 73.1298) (386.2033, 73.4029) (385.7436, 73.9173) (385.5205, 74.6683) (385.5205, 75.1417) knots 0 0 0 1 2 3 4 4 4
  spline S115 degree 2 poles (385.5205, 75.1417) (385.5205, 75.556) (385.7572, 76.2888) (386.2124, 76.8442) (386.8725, 77.1719) (387.2913, 77.1719) knots 0 0 0 1 2 3 4 4 4
  spline S116 degree 2 poles (387.2913, 77.1719) (387.7009, 77.1719) (388.3337, 76.917) (388.7615, 76.4436) (388.9846, 75.7745) (388.9846, 75.3557) knots 0 0 0 1 2 3 4 4 4
  spline S117 degree 2 poles (388.279, 75.4513) (388.2927, 75.7107) (388.1652, 76.1432) (387.9058, 76.4573) (387.5189, 76.6302) (387.2594, 76.6302) knots 0 0 0 1 2 3 4 4 4
  spline S118 degree 2 poles (387.2594, 76.6302) (387.0409, 76.6302) (386.6722, 76.4573) (386.4082, 76.1477) (386.2443, 75.7107) (386.2261, 75.4513) knots 0 0 0 1 2 3 4 4 4
  line L148 (386.2261, 75.4513) -> (388.279, 75.4513)
  line L149 (390.2273, 77.0991) -> (390.8463, 77.0991)
  line L150 (390.8463, 77.0991) -> (390.8646, 76.3799)
  spline S119 degree 2 poles (390.8646, 76.3799) (391.2105, 76.7987) (391.8796, 77.1719) (392.2256, 77.1719) knots 0 0 0 1 2 2 2
  spline S120 degree 2 poles (392.2256, 77.1719) (392.831, 77.1719) (393.4546, 76.3844) (393.4319, 75.6106) knots 0 0 0 1 2 2 2
  line L151 (393.4319, 75.6106) -> (392.7491, 75.6106)
  spline S121 degree 2 poles (392.7491, 75.6106) (392.7627, 76.125) (392.4395, 76.5893) (392.1255, 76.5893) knots 0 0 0 1 2 2 2
  spline S122 degree 2 poles (392.1255, 76.5893) (391.9889, 76.5893) (391.7158, 76.4937) (391.4244, 76.2752) (391.0967, 75.9429) (390.9101, 75.7016) knots 0 0 0 1 2 3 4 4 4
  line L152 (390.9101, 75.7016) -> (390.9101, 73.1981)
  line L153 (390.9101, 73.1981) -> (390.2273, 73.1981)
  line L154 (390.2273, 73.1981) -> (390.2273, 77.0991)
  spline S123 degree 2 poles (397.8427, 75.1827) (397.8427, 74.7275) (397.5878, 73.9673) (397.1053, 73.4302) (396.4134, 73.1298) (395.9719, 73.1298) knots 0 0 0 1 2 3 4 4 4
  spline S124 degree 2 poles (395.9719, 73.1298) (395.5531, 73.1298) (394.8885, 73.3892) (394.4287, 73.8945) (394.1829, 74.641) (394.1829, 75.1281) knots 0 0 0 1 2 3 4 4 4
  spline S125 degree 2 poles (394.1829, 75.1281) (394.1829, 75.5833) (394.4379, 76.3344) (394.9204, 76.8715) (395.6123, 77.1719) (396.0538, 77.1719) knots 0 0 0 1 2 3 4 4 4
  spline S126 degree 2 poles (396.0538, 77.1719) (396.4726, 77.1719) (397.1372, 76.9125) (397.5969, 76.4117) (397.8427, 75.6652) (397.8427, 75.1827) knots 0 0 0 1 2 3 4 4 4
  spline S127 degree 2 poles (397.1508, 75.1509) (397.1508, 75.515) (396.9915, 76.0521) (396.6956, 76.4163) (396.2723, 76.5984) (396.0128, 76.5984) knots 0 0 0 1 2 3 4 4 4
  spline S128 degree 2 poles (396.0128, 76.5984) (395.7079, 76.5984) (395.28, 76.3617) (395.0023, 75.9657) (394.8748, 75.4422) (394.8748, 75.1509) knots 0 0 0 1 2 3 4 4 4
  spline S129 degree 2 poles (394.8748, 75.1509) (394.8748, 74.7912) (395.0342, 74.2496) (395.33, 73.8854) (395.7488, 73.7033) (396.0128, 73.7033) knots 0 0 0 1 2 3 4 4 4
  spline S130 degree 2 poles (396.0128, 73.7033) (396.3178, 73.7033) (396.7457, 73.94) (397.0234, 74.336) (397.1508, 74.8595) (397.1508, 75.1509) knots 0 0 0 1 2 3 4 4 4
  line L155 (398.826, 77.0991) -> (399.4314, 77.0991)
  line L156 (399.4314, 77.0991) -> (399.4587, 76.4709)
  spline S131 degree 2 poles (399.4587, 76.4709) (399.6271, 76.6712) (399.9457, 76.9398) (400.2553, 77.1036) (400.5739, 77.1719) (400.7469, 77.1719) knots 0 0 0 1 2 3 4 4 4
  spline S132 degree 2 poles (400.7469, 77.1719) (401.3477, 77.1719) (401.9668, 76.4618) (401.9668, 75.7472) knots 0 0 0 1 2 2 2
  line L157 (401.9668, 75.7472) -> (401.9668, 73.1981)
  line L158 (401.9668, 73.1981) -> (401.2886, 73.1981)
  line L159 (401.2886, 73.1981) -> (401.2886, 75.6925)
  spline S133 degree 2 poles (401.2886, 75.6925) (401.2886, 76.1477) (400.9472, 76.5893) (400.6103, 76.5893) knots 0 0 0 1 2 2 2
  spline S134 degree 2 poles (400.6103, 76.5893) (400.4829, 76.5893) (400.2462, 76.5164) (399.9913, 76.3344) (399.6908, 76.0203) (399.5042, 75.7881) knots 0 0 0 1 2 3 4 4 4
  line L160 (399.5042, 75.7881) -> (399.5042, 73.1981)
  line L161 (399.5042, 73.1981) -> (398.826, 73.1981)
  line L162 (398.826, 73.1981) -> (398.826, 77.0991)
  line L163 (411.1481, 73.1981) -> (410.4699, 73.1981)
  line L164 (410.4699, 73.1981) -> (410.3698, 76.3708)
  line L165 (410.3698, 76.3708) -> (410.3288, 77.5816)
  line L166 (410.3288, 77.5816) -> (410.0921, 76.876)
  line L167 (410.0921, 76.876) -> (409.341, 74.855)
  line L168 (409.341, 74.855) -> (408.8631, 74.855)
  line L169 (408.8631, 74.855) -> (408.1484, 76.7987)
  line L170 (408.1484, 76.7987) -> (407.9162, 77.5816)
  line L171 (407.9162, 77.5816) -> (407.898, 76.3162)
  line L172 (407.898, 76.3162) -> (407.807, 73.1981)
  line L173 (407.807, 73.1981) -> (407.1561, 73.1981)
  line L174 (407.1561, 73.1981) -> (407.4064, 78.2781)
  line L175 (407.4064, 78.2781) -> (408.2258, 78.2781)
  line L176 (408.2258, 78.2781) -> (408.9086, 76.3662)
  line L177 (408.9086, 76.3662) -> (409.1271, 75.7198)
  line L178 (409.1271, 75.7198) -> (409.341, 76.3662)
  line L179 (409.341, 76.3662) -> (410.0602, 78.2781)
  line L180 (410.0602, 78.2781) -> (410.9023, 78.2781)
  line L181 (410.9023, 78.2781) -> (411.1481, 73.1981)
  line L182 (414.4711, 73.1981) -> (414.4574, 73.7215)
  spline S135 degree 2 poles (414.4574, 73.7215) (414.1388, 73.4074) (413.4787, 73.1298) (413.1191, 73.1298) knots 0 0 0 1 2 2 2
  spline S136 degree 2 poles (413.1191, 73.1298) (412.7823, 73.1298) (412.3089, 73.3028) (412.0039, 73.5986) (411.8582, 74.0038) (411.8582, 74.2405) knots 0 0 0 1 2 3 4 4 4
  spline S137 degree 2 poles (411.8582, 74.2405) (411.8582, 74.8277) (412.7322, 75.4922) (413.588, 75.4922) knots 0 0 0 1 2 2 2
  line L183 (413.588, 75.4922) -> (414.3982, 75.4922)
  line L184 (414.3982, 75.4922) -> (414.3982, 75.8336)
  spline S138 degree 2 poles (414.3982, 75.8336) (414.3982, 76.1796) (413.9567, 76.5984) (413.5015, 76.5984) knots 0 0 0 1 2 2 2
  spline S139 degree 2 poles (413.5015, 76.5984) (413.1692, 76.5984) (412.5274, 76.4527) (412.186, 76.3162) knots 0 0 0 1 2 2 2
  line L185 (412.186, 76.3162) -> (412.186, 76.9261)
  spline S140 degree 2 poles (412.186, 76.9261) (412.3134, 76.9716) (412.6275, 77.0627) (412.978, 77.131) (413.3604, 77.1719) (413.5516, 77.1719) knots 0 0 0 1 2 3 4 4 4
  spline S141 degree 2 poles (413.5516, 77.1719) (413.9066, 77.1719) (414.4756, 77.0172) (414.8671, 76.6985) (415.0765, 76.216) (415.0765, 75.8883) knots 0 0 0 1 2 3 4 4 4
  line L186 (415.0765, 75.8883) -> (415.0765, 73.1981)
  line L187 (415.0765, 73.1981) -> (414.4711, 73.1981)
  line L188 (414.3982, 74.9733) -> (413.5379, 74.9733)
  spline S142 degree 2 poles (413.5379, 74.9733) (413.283, 74.9733) (412.9189, 74.8732) (412.6867, 74.6865) (412.5729, 74.4271) (412.5729, 74.2632) knots 0 0 0 1 2 3 4 4 4
  spline S143 degree 2 poles (412.5729, 74.2632) (412.5729, 74.1494) (412.6412, 73.9446) (412.8005, 73.7853) (413.0463, 73.6942) (413.2284, 73.6942) knots 0 0 0 1 2 3 4 4 4
  spline S144 degree 2 poles (413.2284, 73.6942) (413.4605, 73.6942) (414.0614, 73.9764) (414.3982, 74.2814) knots 0 0 0 1 2 2 2
  line L189 (414.3982, 74.2814) -> (414.3982, 74.9733)
  line L190 (416.5013, 77.0991) -> (417.1203, 77.0991)
  line L191 (417.1203, 77.0991) -> (417.1385, 76.3799)
  spline S145 degree 2 poles (417.1385, 76.3799) (417.4845, 76.7987) (418.1536, 77.1719) (418.4996, 77.1719) knots 0 0 0 1 2 2 2
  spline S146 degree 2 poles (418.4996, 77.1719) (419.105, 77.1719) (419.7286, 76.3844) (419.7058, 75.6106) knots 0 0 0 1 2 2 2
  line L192 (419.7058, 75.6106) -> (419.0231, 75.6106)
  spline S147 degree 2 poles (419.0231, 75.6106) (419.0367, 76.125) (418.7135, 76.5893) (418.3994, 76.5893) knots 0 0 0 1 2 2 2
  spline S148 degree 2 poles (418.3994, 76.5893) (418.2629, 76.5893) (417.9898, 76.4937) (417.6984, 76.2752) (417.3707, 75.9429) (417.1841, 75.7016) knots 0 0 0 1 2 3 4 4 4
  line L193 (417.1841, 75.7016) -> (417.1841, 73.1981)
  line L194 (417.1841, 73.1981) -> (416.5013, 73.1981)
  line L195 (416.5013, 73.1981) -> (416.5013, 77.0991)
  line L196 (424.226, 73.1981) -> (423.2974, 73.1981)
  line L197 (423.2974, 73.1981) -> (421.4811, 75.292)
  line L198 (421.4811, 75.292) -> (421.4811, 73.1981)
  line L199 (421.4811, 73.1981) -> (420.8029, 73.1981)
  line L200 (420.8029, 73.1981) -> (420.8029, 78.6923)
  line L201 (420.8029, 78.6923) -> (421.4811, 78.6923)
  line L202 (421.4811, 78.6923) -> (421.4811, 75.3193)
  line L203 (421.4811, 75.3193) -> (423.2336, 77.0991)
  line L204 (423.2336, 77.0991) -> (424.1258, 77.0991)
  line L205 (424.1258, 77.0991) -> (422.2959, 75.3011)
  line L206 (422.2959, 75.3011) -> (424.226, 73.1981)
  line L207 (428.2408, 73.1981) -> (427.5625, 73.1981)
  line L208 (427.5625, 73.1981) -> (427.5625, 75.6925)
  spline S149 degree 2 poles (427.5625, 75.6925) (427.5625, 76.1432) (427.2257, 76.5893) (426.9116, 76.5893) knots 0 0 0 1 2 2 2
  spline S150 degree 2 poles (426.9116, 76.5893) (426.7751, 76.5893) (426.5384, 76.5164) (426.2789, 76.3344) (425.9785, 76.0203) (425.7782, 75.7881) knots 0 0 0 1 2 3 4 4 4
  line L209 (425.7782, 75.7881) -> (425.7782, 73.1981)
  line L210 (425.7782, 73.1981) -> (425.0999, 73.1981)
  line L211 (425.0999, 73.1981) -> (425.0999, 78.6923)
  line L212 (425.0999, 78.6923) -> (425.7782, 78.6923)
  line L213 (425.7782, 78.6923) -> (425.7782, 77.1036)
  line L214 (425.7782, 77.1036) -> (425.7554, 76.4891)
  spline S151 degree 2 poles (425.7554, 76.4891) (425.9147, 76.6803) (426.2197, 76.9398) (426.5293, 77.1036) (426.8479, 77.1719) (427.0209, 77.1719) knots 0 0 0 1 2 3 4 4 4
  spline S152 degree 2 poles (427.0209, 77.1719) (427.6035, 77.1719) (428.2408, 76.4618) (428.2408, 75.7472) knots 0 0 0 1 2 2 2
  line L215 (428.2408, 75.7472) -> (428.2408, 73.1981)
  line L216 (431.9871, 73.1981) -> (431.9734, 73.7215)
  spline S153 degree 2 poles (431.9734, 73.7215) (431.6548, 73.4074) (430.9947, 73.1298) (430.6351, 73.1298) knots 0 0 0 1 2 2 2
  spline S154 degree 2 poles (430.6351, 73.1298) (430.2983, 73.1298) (429.8249, 73.3028) (429.5199, 73.5986) (429.3742, 74.0038) (429.3742, 74.2405) knots 0 0 0 1 2 3 4 4 4
  spline S155 degree 2 poles (429.3742, 74.2405) (429.3742, 74.8277) (430.2482, 75.4922) (431.104, 75.4922) knots 0 0 0 1 2 2 2
  line L217 (431.104, 75.4922) -> (431.9142, 75.4922)
  line L218 (431.9142, 75.4922) -> (431.9142, 75.8336)
  spline S156 degree 2 poles (431.9142, 75.8336) (431.9142, 76.1796) (431.4727, 76.5984) (431.0175, 76.5984) knots 0 0 0 1 2 2 2
  spline S157 degree 2 poles (431.0175, 76.5984) (430.6852, 76.5984) (430.0434, 76.4527) (429.702, 76.3162) knots 0 0 0 1 2 2 2
  line L219 (429.702, 76.3162) -> (429.702, 76.9261)
  spline S158 degree 2 poles (429.702, 76.9261) (429.8294, 76.9716) (430.1435, 77.0627) (430.494, 77.131) (430.8764, 77.1719) (431.0676, 77.1719) knots 0 0 0 1 2 3 4 4 4
  spline S159 degree 2 poles (431.0676, 77.1719) (431.4226, 77.1719) (431.9916, 77.0172) (432.3831, 76.6985) (432.5925, 76.216) (432.5925, 75.8883) knots 0 0 0 1 2 3 4 4 4
  line L220 (432.5925, 75.8883) -> (432.5925, 73.1981)
  line L221 (432.5925, 73.1981) -> (431.9871, 73.1981)
  line L222 (431.9142, 74.9733) -> (431.0539, 74.9733)
  spline S160 degree 2 poles (431.0539, 74.9733) (430.799, 74.9733) (430.4348, 74.8732) (430.2027, 74.6865) (430.0889, 74.4271) (430.0889, 74.2632) knots 0 0 0 1 2 3 4 4 4
  spline S161 degree 2 poles (430.0889, 74.2632) (430.0889, 74.1494) (430.1572, 73.9446) (430.3165, 73.7853) (430.5623, 73.6942) (430.7444, 73.6942) knots 0 0 0 1 2 3 4 4 4
  spline S162 degree 2 poles (430.7444, 73.6942) (430.9765, 73.6942) (431.5774, 73.9764) (431.9142, 74.2814) knots 0 0 0 1 2 2 2
  line L223 (431.9142, 74.2814) -> (431.9142, 74.9733)
  line L224 (436.6437, 73.1981) -> (436.6437, 76.0021)
  spline S163 degree 2 poles (436.6437, 76.0021) (436.6437, 76.1841) (436.6164, 76.4163) (436.5618, 76.5529) (436.4799, 76.6075) (436.4161, 76.6075) knots 0 0 0 1 2 3 4 4 4
  spline S164 degree 2 poles (436.4161, 76.6075) (436.3433, 76.6075) (436.2204, 76.5164) (436.0793, 76.3025) (435.9109, 75.9565) (435.7925, 75.7062) knots 0 0 0 1 2 3 4 4 4
  line L225 (435.7925, 75.7062) -> (435.7925, 73.1981)
  line L226 (435.7925, 73.1981) -> (435.1143, 73.1981)
  line L227 (435.1143, 73.1981) -> (435.1143, 75.9292)
  spline S165 degree 2 poles (435.1143, 75.9292) (435.1143, 76.1432) (435.087, 76.4072) (435.0323, 76.5529) (434.9458, 76.6075) (434.8821, 76.6075) knots 0 0 0 1 2 3 4 4 4
  spline S166 degree 2 poles (434.8821, 76.6075) (434.8184, 76.6075) (434.7, 76.5301) (434.5589, 76.3298) (434.3814, 75.9793) (434.2631, 75.7062) knots 0 0 0 1 2 3 4 4 4
  line L228 (434.2631, 75.7062) -> (434.2631, 73.1981)
  line L229 (434.2631, 73.1981) -> (433.5848, 73.1981)
  line L230 (433.5848, 73.1981) -> (433.5848, 77.0991)
  line L231 (433.5848, 77.0991) -> (434.1493, 77.0991)
  line L232 (434.1493, 77.0991) -> (434.1811, 76.3571)
  spline S167 degree 2 poles (434.1811, 76.3571) (434.2858, 76.5802) (434.477, 76.8897) (434.6773, 77.0809) (434.9094, 77.1719) (435.046, 77.1719) knots 0 0 0 1 2 3 4 4 4
  spline S168 degree 2 poles (435.046, 77.1719) (435.3646, 77.1719) (435.6924, 76.7577) (435.6924, 76.3253) knots 0 0 0 1 2 2 2
  spline S169 degree 2 poles (435.6924, 76.3253) (435.7834, 76.5301) (435.9655, 76.8442) (436.1703, 77.0581) (436.4207, 77.1719) (436.5846, 77.1719) knots 0 0 0 1 2 3 4 4 4
  spline S170 degree 2 poles (436.5846, 77.1719) (437.322, 77.1719) (437.322, 76.0385) knots 0 0 0 1 1 1
  line L233 (437.322, 76.0385) -> (437.322, 73.1981)
  line L234 (437.322, 73.1981) -> (436.6437, 73.1981)
  spline S171 degree 2 poles (323.3315, 68.1555) (323.3315, 67.8459) (323.0994, 67.236) (322.6077, 66.7535) (321.8476, 66.453) (321.315, 66.453) knots 0 0 0 1 2 3 4 4 4
  line L235 (321.315, 66.453) -> (320.6868, 66.453)
  line L236 (320.6868, 66.453) -> (320.6868, 64.6322)
  line L237 (320.6868, 64.6322) -> (319.9949, 64.6322)
  line L238 (319.9949, 64.6322) -> (319.9949, 69.7122)
  line L239 (319.9949, 69.7122) -> (321.4242, 69.7122)
  spline S172 degree 2 poles (321.4242, 69.7122) (321.802, 69.7122) (322.4939, 69.5438) (323.022, 69.1706) (323.3315, 68.5788) (323.3315, 68.1555) knots 0 0 0 1 2 3 4 4 4
  spline S173 degree 2 poles (322.6123, 68.1282) (322.6123, 68.6152) (321.9705, 69.1387) (321.3969, 69.1387) knots 0 0 0 1 2 2 2
  line L240 (321.3969, 69.1387) -> (320.6868, 69.1387)
  line L241 (320.6868, 69.1387) -> (320.6868, 67.0448)
  line L242 (320.6868, 67.0448) -> (321.3332, 67.0448)
  spline S174 degree 2 poles (321.3332, 67.0448) (321.9477, 67.0448) (322.6123, 67.5819) (322.6123, 68.1282) knots 0 0 0 1 2 2 2
  spline S175 degree 2 poles (327.7788, 66.6169) (327.7788, 66.1617) (327.5239, 65.4015) (327.0414, 64.8644) (326.3495, 64.564) (325.9079, 64.564) knots 0 0 0 1 2 3 4 4 4
  spline S176 degree 2 poles (325.9079, 64.564) (325.4891, 64.564) (324.8246, 64.8234) (324.3648, 65.3287) (324.119, 66.0752) (324.119, 66.5623) knots 0 0 0 1 2 3 4 4 4
  spline S177 degree 2 poles (324.119, 66.5623) (324.119, 67.0175) (324.3739, 67.7686) (324.8564, 68.3057) (325.5483, 68.6061) (325.9899, 68.6061) knots 0 0 0 1 2 3 4 4 4
  spline S178 degree 2 poles (325.9899, 68.6061) (326.4086, 68.6061) (327.0732, 68.3467) (327.533, 67.8459) (327.7788, 67.0994) (327.7788, 66.6169) knots 0 0 0 1 2 3 4 4 4
  spline S179 degree 2 poles (327.0869, 66.585) (327.0869, 66.9492) (326.9276, 67.4863) (326.6317, 67.8505) (326.2084, 68.0326) (325.9489, 68.0326) knots 0 0 0 1 2 3 4 4 4
  spline S180 degree 2 poles (325.9489, 68.0326) (325.6439, 68.0326) (325.216, 67.7959) (324.9384, 67.3998) (324.8109, 66.8764) (324.8109, 66.585) knots 0 0 0 1 2 3 4 4 4
  spline S181 degree 2 poles (324.8109, 66.585) (324.8109, 66.2254) (324.9702, 65.6837) (325.2661, 65.3196) (325.6849, 65.1375) (325.9489, 65.1375) knots 0 0 0 1 2 3 4 4 4
  spline S182 degree 2 poles (325.9489, 65.1375) (326.2539, 65.1375) (326.6818, 65.3742) (326.9594, 65.7702) (327.0869, 66.2937) (327.0869, 66.585) knots 0 0 0 1 2 3 4 4 4
  line L243 (332.3763, 68.5333) -> (331.8073, 64.6322)
  line L244 (331.8073, 64.6322) -> (330.9879, 64.6322)
  line L245 (330.9879, 64.6322) -> (330.4235, 66.2664)
  line L246 (330.4235, 66.2664) -> (330.3142, 66.6624)
  line L247 (330.3142, 66.6624) -> (330.1822, 66.2436)
  line L248 (330.1822, 66.2436) -> (329.6405, 64.6322)
  line L249 (329.6405, 64.6322) -> (328.8439, 64.6322)
  line L250 (328.8439, 64.6322) -> (328.2841, 68.5333)
  line L251 (328.2841, 68.5333) -> (328.9441, 68.5333)
  line L252 (328.9441, 68.5333) -> (329.2673, 65.884)
  line L253 (329.2673, 65.884) -> (329.3401, 65.2923)
  line L254 (329.3401, 65.2923) -> (329.504, 65.8067)
  line L255 (329.504, 65.8067) -> (330.073, 67.5637)
  line L256 (330.073, 67.5637) -> (330.56, 67.5637)
  line L257 (330.56, 67.5637) -> (331.17, 65.8294)
  line L258 (331.17, 65.8294) -> (331.3475, 65.315)
  line L259 (331.3475, 65.315) -> (331.4022, 65.8613)
  line L260 (331.4022, 65.8613) -> (331.7071, 68.5333)
  line L261 (331.7071, 68.5333) -> (332.3763, 68.5333)
  spline S183 degree 2 poles (336.4366, 66.7899) (336.4366, 66.6488) (336.4275, 66.453) (336.423, 66.3665) knots 0 0 0 1 2 2 2
  line L262 (336.423, 66.3665) -> (333.6781, 66.3665)
  spline S184 degree 2 poles (333.6781, 66.3665) (333.6781, 65.7702) (334.3473, 65.1284) (334.98, 65.1284) knots 0 0 0 1 2 2 2
  spline S185 degree 2 poles (334.98, 65.1284) (335.1484, 65.1284) (335.4898, 65.1557) (335.813, 65.2012) (336.1043, 65.2604) (336.2272, 65.2968) knots 0 0 0 1 2 3 4 4 4
  line L263 (336.2272, 65.2968) -> (336.2272, 64.7415)
  spline S186 degree 2 poles (336.2272, 64.7415) (335.9496, 64.6641) (335.2531, 64.564) (334.8799, 64.564) knots 0 0 0 1 2 2 2
  spline S187 degree 2 poles (334.8799, 64.564) (334.3791, 64.564) (333.6554, 64.8371) (333.1956, 65.3515) (332.9726, 66.1025) (332.9726, 66.5759) knots 0 0 0 1 2 3 4 4 4
  spline S188 degree 2 poles (332.9726, 66.5759) (332.9726, 66.9902) (333.2093, 67.723) (333.6645, 68.2784) (334.3245, 68.6061) (334.7433, 68.6061) knots 0 0 0 1 2 3 4 4 4
  spline S189 degree 2 poles (334.7433, 68.6061) (335.153, 68.6061) (335.7857, 68.3512) (336.2136, 67.8778) (336.4366, 67.2087) (336.4366, 66.7899) knots 0 0 0 1 2 3 4 4 4
  spline S190 degree 2 poles (335.7311, 66.8855) (335.7447, 67.1449) (335.6173, 67.5774) (335.3578, 67.8915) (334.9709, 68.0644) (334.7114, 68.0644) knots 0 0 0 1 2 3 4 4 4
  spline S191 degree 2 poles (334.7114, 68.0644) (334.4929, 68.0644) (334.1242, 67.8915) (333.8602, 67.5819) (333.6963, 67.1449) (333.6781, 66.8855) knots 0 0 0 1 2 3 4 4 4
  line L264 (333.6781, 66.8855) -> (335.7311, 66.8855)
  line L265 (337.6793, 68.5333) -> (338.2984, 68.5333)
  line L266 (338.2984, 68.5333) -> (338.3166, 67.8141)
  spline S192 degree 2 poles (338.3166, 67.8141) (338.6625, 68.2329) (339.3317, 68.6061) (339.6776, 68.6061) knots 0 0 0 1 2 2 2
  spline S193 degree 2 poles (339.6776, 68.6061) (340.283, 68.6061) (340.9067, 67.8186) (340.8839, 67.0448) knots 0 0 0 1 2 2 2
  line L267 (340.8839, 67.0448) -> (340.2011, 67.0448)
  spline S194 degree 2 poles (340.2011, 67.0448) (340.2148, 67.5592) (339.8916, 68.0235) (339.5775, 68.0235) knots 0 0 0 1 2 2 2
  spline S195 degree 2 poles (339.5775, 68.0235) (339.4409, 68.0235) (339.1678, 67.9279) (338.8765, 67.7094) (338.5487, 67.3771) (338.3621, 67.1358) knots 0 0 0 1 2 3 4 4 4
  line L268 (338.3621, 67.1358) -> (338.3621, 64.6322)
  line L269 (338.3621, 64.6322) -> (337.6793, 64.6322)
  line L270 (337.6793, 64.6322) -> (337.6793, 68.5333)
  spline S196 degree 2 poles (345.1946, 66.7899) (345.1946, 66.6488) (345.1855, 66.453) (345.181, 66.3665) knots 0 0 0 1 2 2 2
  line L271 (345.181, 66.3665) -> (342.4361, 66.3665)
  spline S197 degree 2 poles (342.4361, 66.3665) (342.4361, 65.7702) (343.1053, 65.1284) (343.738, 65.1284) knots 0 0 0 1 2 2 2